Autodesk Inventor part; units mm, degrees
(part 2 of 2)
  spline S260 degree 2 poles (-11.6657, -29.851) (-11.6657, -29.7809) (-11.7541, -29.6726) (-11.8684, -29.6422) knots 0 0 0 1 2 2 2
  spline S261 degree 2 poles (-11.8684, -29.6422) (-12.0163, -29.6025) (-12.3684, -29.6025) knots 0 0 0 1 1 1
  spline S262 degree 2 poles (-12.3684, -29.6025) (-12.719, -29.6025) (-12.9827, -29.6742) (-13.0696, -29.7809) (-13.0696, -29.851) knots 0 0 0 1 2 3 3 3
  spline S263 degree 2 poles (-13.0696, -29.851) (-13.0696, -29.9211) (-12.9812, -30.0294) (-12.8669, -30.0598) knots 0 0 0 1 2 2 2
  spline S264 degree 2 poles (-12.8669, -30.0598) (-12.719, -30.0995) (-12.3684, -30.0995) knots 0 0 0 1 1 1
  spline S265 degree 2 poles (-12.3684, -30.0995) (-12.0163, -30.0995) (-11.7541, -30.0278) (-11.6657, -29.9211) (-11.6657, -29.851) knots 0 0 0 1 2 3 3 3
  line L189 (-12.998, -32.0507) -> (-13.3547, -32.0507)
  line L190 (-13.3547, -32.0507) -> (-13.3547, -30.7077)
  spline S266 degree 2 poles (-13.3547, -30.7077) (-13.1535, -30.729) (-12.7922, -30.947) (-12.4934, -31.2702) knots 0 0 0 1 2 2 2
  spline S267 degree 2 poles (-12.4934, -31.2702) (-12.2526, -31.5294) (-12.1657, -31.5873) knots 0 0 0 1 1 1
  spline S268 degree 2 poles (-12.1657, -31.5873) (-12.0468, -31.6665) (-11.9309, -31.6665) knots 0 0 0 1 1 1
  spline S269 degree 2 poles (-11.9309, -31.6665) (-11.8029, -31.6665) (-11.6657, -31.5294) (-11.6657, -31.4074) knots 0 0 0 1 2 2 2
  spline S270 degree 2 poles (-11.6657, -31.4074) (-11.6657, -31.2885) (-11.8105, -31.1467) (-11.9782, -31.1361) knots 0 0 0 1 2 2 2
  line L191 (-11.9782, -31.1361) -> (-11.9401, -30.7534)
  spline S271 degree 2 poles (-11.9401, -30.7534) (-11.623, -30.787) (-11.3471, -31.1467) (-11.3471, -31.4165) knots 0 0 0 1 2 2 2
  spline S272 degree 2 poles (-11.3471, -31.4165) (-11.3471, -31.7123) (-11.6657, -32.0507) (-11.9035, -32.0507) knots 0 0 0 1 2 2 2
  spline S273 degree 2 poles (-11.9035, -32.0507) (-12.0376, -32.0507) (-12.2815, -31.9547) (-12.4157, -31.8495) knots 0 0 0 1 2 2 2
  spline S274 degree 2 poles (-12.4157, -31.8495) (-12.5041, -31.7794) (-12.8364, -31.4165) (-12.9462, -31.319) (-12.998, -31.29) knots 0 0 0 1 2 3 3 3
  line L192 (-12.998, -31.29) -> (-12.998, -32.0507)
  line L193 (-12.8227, -32.2961) -> (-12.777, -32.6665)
  spline S275 degree 2 poles (-12.777, -32.6665) (-12.9187, -32.6848) (-13.0696, -32.8403) (-13.0696, -32.9501) knots 0 0 0 1 2 2 2
  spline S276 degree 2 poles (-13.0696, -32.9501) (-13.0696, -33.069) (-12.8898, -33.2306) (-12.7373, -33.2306) knots 0 0 0 1 2 2 2
  spline S277 degree 2 poles (-12.7373, -33.2306) (-12.5925, -33.2306) (-12.4233, -33.0766) (-12.4233, -32.9653) knots 0 0 0 1 2 2 2
  spline S278 degree 2 poles (-12.4233, -32.9653) (-12.4233, -32.8922) (-12.4523, -32.79) knots 0 0 0 1 1 1
  line L194 (-12.4523, -32.79) -> (-12.1398, -32.8327)
  spline S279 degree 2 poles (-12.1398, -32.8327) (-12.1443, -32.9882) (-12.001, -33.1513) (-11.8821, -33.1513) knots 0 0 0 1 2 2 2
  spline S280 degree 2 poles (-11.8821, -33.1513) (-11.7815, -33.1513) (-11.6626, -33.0309) (-11.6626, -32.9318) knots 0 0 0 1 2 2 2
  spline S281 degree 2 poles (-11.6626, -32.9318) (-11.6626, -32.8327) (-11.7983, -32.694) (-11.9294, -32.6787) knots 0 0 0 1 2 2 2
  line L195 (-11.9294, -32.6787) -> (-11.8699, -32.3251)
  spline S282 degree 2 poles (-11.8699, -32.3251) (-11.6885, -32.3617) (-11.4706, -32.5111) (-11.3471, -32.7763) (-11.3471, -32.9425) knots 0 0 0 1 2 3 3 3
  spline S283 degree 2 poles (-11.3471, -32.9425) (-11.3471, -33.2245) (-11.527, -33.3952) knots 0 0 0 1 1 1
  spline S284 degree 2 poles (-11.527, -33.3952) (-11.6733, -33.5354) (-11.8593, -33.5354) knots 0 0 0 1 1 1
  spline S285 degree 2 poles (-11.8593, -33.5354) (-12.1215, -33.5354) (-12.2785, -33.2473) knots 0 0 0 1 1 1
  spline S286 degree 2 poles (-12.2785, -33.2473) (-12.3151, -33.4196) (-12.5727, -33.6239) (-12.7541, -33.6239) knots 0 0 0 1 2 2 2
  spline S287 degree 2 poles (-12.7541, -33.6239) (-13.0178, -33.6239) (-13.3882, -33.2397) (-13.3882, -32.9531) knots 0 0 0 1 2 2 2
  spline S288 degree 2 poles (-13.3882, -32.9531) (-13.3882, -32.6818) (-13.0757, -32.3251) (-12.8227, -32.2961) knots 0 0 0 1 2 2 2
  point P0 (0, 0)
  constraints: 2 other
extrude "Extrusion14" cut sketch "Sketch10" against normal blind 0.5
body "Solid6"
